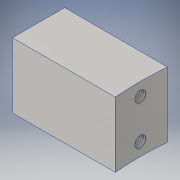
# Autodesk Inventor part: mountingStub
Saved by Autodesk Inventor 2016 SP1 (Build 200210100, 210)
## iProperties
Created: 2015-12-10
Part Number: mountingStub
Material: Aluminum 6061
Document SubType Name: Modeling
Designer: Dave
Density: 2.7 g/cm^3
Appearance: Aluminum - Flat
Mass: 149.9 g
Surface Area: 113.278 cm^2
Volume: 55.5184 cm^3
Author: Dave
Autodesk Inventor part; units mm, degrees
ref_plane "YZ Plane" through (0, 0, 0) normal (1, 0, 0) x (0, 1, 0)
ref_plane "XZ Plane" through (0, 0, 0) normal (0, 1, 0) x (-1, 0, 0)
ref_plane "XY Plane" through (0, 0, 0) normal (0, 0, 1) x (1, 0, 0)
sketch "Sketch1" plane through (0, 0, 0) normal (0, 1, 0) x (-1, 0, 0)
  line L0 (0, 0) -> (50.8, 0)
  line L1 (50.8, 0) -> (50.8, -25.4)
  line L2 (50.8, -25.4) -> (0, -25.4)
  line L3 (0, -25.4) -> (0, 0)
  dimension "d0" = 25.4
  dimension "d1" = 50.8
  constraints: 8 end point, 2 parallel, 1 horizontal, 1 perpendicular
  measures "d0" distance of L2.end L0.start
  measures "d1" distance of L0.start L0.end
extrude "Extrusion1" add sketch "Sketch1" along normal blind 31.75
sketch "Sketch3" plane through (0, 0, 0) normal (1, 0, 0) x (0, 0, -1)
  circle A0 centre (12.7, 25.4) radius 2.581
  line L0 (0, 31.75) -> (25.4, 31.75) projected
  circle A1 centre (12.7, 6.35) radius 2.3807
  point P0 (0, 0)
  dimension "d6" = 6.35
  dimension "d7" = 19.05
  constraints: 2 centre point
  measures "d6" distance from line of A0.centre L0
  measures "d7" distance of A1.centre A0.centre
hole "Hole1" at (0, 25.4, -12.7) at (0, 6.35, -12.7) direction (-1, 0, 0) diameter 5.3594 depth 17.2466 tip angle 118 thread size "1/4-28 UNF" class "2B" standard "ANSI Unified Screw Threads"
sketch "Sketch4" plane through (0, 31.75, 0) normal (0, 1, 0) x (1, 0, 0)
  line L0 (0, 0) -> (0, 25.4) projected
  line L1 (0, 12.7) -> (146.05, 12.7) construction
  circle A0 centre (146.05, 12.7) radius 147.32
  dimension "d15" = 146.05
  dimension "d16" = 294.64
  constraints: 2 end point, 1 centre point, 1 coincident, 1 horizontal, 1 midpoint
  measures "d15" distance of L1.start L1.end
  measures "d16" diameter of A0
extrude "Extrusion2" cut sketch "Sketch4" against normal blind 50.8
sketch "Sketch6" plane through (0, 0, 0) normal (0, -1, 0) x (1, 0, 0)
  circle A0 centre (-44.45, -12.7) radius 4.2294
  line L0 (-0.7216, 0) -> (-50.8, 0) projected
  line L1 (-50.8, 0) -> (-50.8, -25.4) projected
  circle A1 centre (-25.4, -12.7) radius 3.8351
  point P0 (0, 0)
  dimension "d21" = 12.7
  dimension "d22" = 6.35
  dimension "d23" = 19.05
  constraints: 2 centre point
  measures "d21" distance from line of A0.centre L0
  measures "d22" distance from line of A0.centre L1
  measures "d23" distance of A1.centre A0.centre
hole "Hole2" at (-44.45, 0, -12.7) at (-25.4, 0, -12.7) direction (0, 1, 0) diameter 5.3594 depth 17.2466 tip angle 118 thread size "1/4-28 UNF" class "2B" standard "ANSI Unified Screw Threads"
body "Solid1"
